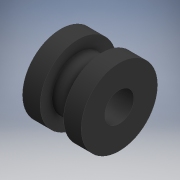
# Autodesk Inventor part: Rubber_Grommet_5mmIDx13mmODx10mm_LM1046
Saved by Autodesk Inventor 2020.3 (Build 243373000, 373)
## iProperties
Created: 2020-05-12
Part Number: Rubber_Grommet_5mmIDx13mmODx10mm_LM1046
Material: Rubber
Document SubType Name: Modeling
Designer: rah75
Density: 0.93 g/cm^3
Appearance: Rubber - Black
Author: rah75
Autodesk Inventor part; units mm, degrees
ref_plane "YZ Plane" through (0, 0, 0) normal (1, 0, 0) x (0, 1, 0)
ref_plane "XZ Plane" through (0, 0, 0) normal (0, 1, 0) x (-1, 0, 0)
ref_plane "XY Plane" through (0, 0, 0) normal (0, 0, 1) x (1, 0, 0)
sketch "Sketch1" plane through (0, 0, 0) normal (0, 0, 1) x (1, 0, 0)
  line L0 (-5, 2.5) -> (5, 2.5)
  line L1 (5, 2.5) -> (5, 6.5)
  line L2 (5, 6.5) -> (2, 6.5)
  line L3 (2, 6.5) -> (2, 4.5)
  line L4 (2, 4.5) -> (-2, 4.5)
  line L5 (-2, 4.5) -> (-2, 6.5)
  line L6 (-2, 6.5) -> (-5, 6.5)
  line L7 (-5, 6.5) -> (-5, 2.5)
  line L8 (0, 0) -> (1.4563, 0)
  point P0 (0, 2.5)
  dimension "d0" = 5
  dimension "d1" = 10
  dimension "d2" = 3
  dimension "d3" = 3
  dimension "d4" = 13
  dimension "d5" = 9
  constraints: 18 end point, 6 perpendicular, 2 horizontal, 2 point on line, 1 midpoint, 1 vertical alignment
  measures "d0" diameter of L0 L8
  measures "d1" distance of L0.start L0.end
  measures "d2" distance of L5.end L6.end
  measures "d3" distance of L1.end L2.end
  measures "d4" diameter of L2 L8
  measures "d5" diameter of L4 L8
revolve "Revolution1" add sketch "Sketch1" angle 360 about axis through (0, 0, 0) along (1, 0, 0)
body "Solid1"
